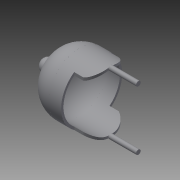
# Autodesk Inventor part: DMJ_hat
Saved by Autodesk Inventor 2015 SP1 (Build 190203100, 203)
## iProperties
Created: 2016-02-03
Part Number: DMJ_hat
Material: Generic
Document SubType Name: Modeling
Designer: guillemd
Density: 1 g/cm^3
Appearance: Default
Author: guillemd
Autodesk Inventor part; units mm, degrees
ref_plane "YZ Plane" through (0, 0, 0) normal (1, 0, 0) x (0, 1, 0)
ref_plane "XZ Plane" through (0, 0, 0) normal (0, 1, 0) x (-1, 0, 0)
ref_plane "XY Plane" through (0, 0, 0) normal (0, 0, 1) x (1, 0, 0)
sketch "Sketch1" plane through (0, 0, 0) normal (0, 1, 0) x (-1, 0, 0)
  line L0 (0, 0) -> (0, 12.7)
  arc A0 (0, 12.7) -> (-64.77, 77.47) centre (-64.77, 12.7) ccw
  line L1 (0, 0) -> (38.1, 0)
  line L2 (-64.77, 77.47) -> (-152.4, 77.47)
  line L3 (-152.4, 77.47) -> (-152.4, 83.82)
  line L4 (-152.4, 83.82) -> (-64.77, 83.82)
  arc A1 (6.35, 12.7) -> (-64.77, 83.82) centre (-64.77, 12.7) ccw
  arc A2 (38.1, 0) -> (6.35, 12.7) centre (19.685, 0) ccw
  line L5 (81.359, 0) -> (-191.3598, 0) projected
  dimension "d0" = 12.7
  dimension "d4" = 152.4
  dimension "d5" = 77.47
  dimension "d6" = 6.35
  dimension "d7" = 12.7
  dimension "d9" = 38.1
  constraints: 10 end point, 6 point on circle, 3 centre point, 2 coincident, 2 horizontal, 2 tangent, 2 vertical, 1 line through centre, 1 parallel, 1 perpendicular
  measures "d0" distance of L0.start L0.end
  measures "d4" horizontal distance of L2.end L0.start
  measures "d5" vertical distance of L0.start L2.end
  measures "d6" distance of L2.end L3.end
  measures "d7" vertical distance of point (0, 0) A1.start
  measures "d9" distance of point (0, 0) L1.end
revolve "Revolution1" add sketch "Sketch1" angle 360 about axis through (-10, 0, 0) along (1, 0, 0)
sketch "Sketch3" plane through (0, 0, 0) normal (0, 1, 0) x (-1, 0, 0)
  line L0 (-99.1769, -83.82) -> (-99.1769, -49.0516)
  line L1 (-99.1769, 83.82) -> (-99.1769, 47.9401)
  line L2 (-152.4, -83.82) -> (-152.4, 83.82)
  line L3 (-99.1769, -49.0516) -> (-124.5769, -49.0516)
  line L4 (-99.1769, 47.9401) -> (-124.5769, 47.9401)
  line L5 (-152.4, -83.82) -> (-64.77, -83.82) projected
  line L6 (-152.4, 83.82) -> (-64.77, 83.82) projected
  line L7 (-99.1769, -83.82) -> (-152.4, -83.82)
  line L8 (-152.4, 83.82) -> (-99.1769, 83.82)
  line L9 (-152.4, -83.82) -> (-152.4, 83.82)
  line L10 (-151.13, -9.525) -> (-151.13, 9.525)
  line L11 (76.2, 0) -> (-190.5, 0) projected
  arc A0 (-151.13, -9.525) -> (-124.5769, -49.0516) centre (-108.4341, -9.525) ccw
  arc A1 (-124.5769, 47.9401) -> (-151.13, 9.525) centre (-110.0654, 9.525) ccw
  point P0 (0, 0)
  point P1 (-152.4, 0)
  point P2 (-151.13, 0)
  dimension "d14" = 25.4
  dimension "d15" = 25.4
  dimension "d18" = 34.7684
  dimension "d22" = 53.2231
  dimension "d23" = 35.8799
  dimension "d26" = 19.05
  dimension "d27" = 1.27
  constraints: 18 end point, 4 point on circle, 3 collinear, 3 point on line, 3 vertical, 2 centre point, 2 horizontal, 2 midpoint, 2 tangent, 1 parallel
  measures "d14" distance of L0.end L3.end
  measures "d15" distance of L1.end L4.end
  measures "d18" distance of L0.start L0.end
  measures "d22" distance of L2.start L0.start
  measures "d23" distance of L1.start L1.end
  measures "d26" distance of L10.start L10.end
  measures "d27" distance between parallel lines of L2 L10
extrude "Extrusion1" cut sketch "Sketch3" along normal through all both and the other way through all
sketch "Sketch4" plane through (151.13, -83.277, -9.525) normal (1, 0, 0) x (0, 0, -1)
  arc A0 (-19.05, 6.3948) -> (0, 6.3948) centre (-9.525, 83.277) ccw projected
  arc A1 (-19.05, 0) -> (0, 0) centre (-9.525, 83.277) ccw projected
  circle A2 centre (-9.525, 1.994) radius 6.35
  arc A3 (0, 160.1593) -> (-19.05, 160.1593) centre (-9.525, 83.277) ccw projected
  arc A4 (0, 166.5541) -> (-19.05, 166.5541) centre (-9.525, 83.277) ccw projected
  circle A5 centre (-9.525, 164.557) radius 6.35
  point P0 (-9.525, 160.747)
  dimension "d28" = 12.7
  dimension "d30" = 81.2831
  dimension "d31" = 12.7
  dimension "d32" = 81.28
  constraints: 2 centre point, 2 vertical alignment, 1 point on circle
  measures "d28" diameter of A2
  measures "d30" distance of point (-9.525, 83.277) A2.centre
  measures "d31" diameter of A5
  measures "d32" distance of A5.centre point (-9.525, 83.277)
extrude "Extrusion2" add sketch "Sketch4" along normal blind 76.2
body "Solid1"
